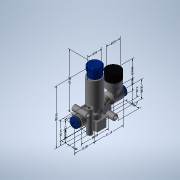
# Autodesk Inventor part: 8086003 VRPA-CM-Q4-E---(0_high)
Saved by Autodesk Inventor 2021 (Build 250183000, 183)
## iProperties
Created: 2026-04-20
Part Number: 8086003 VRPA-CM-Q4-E---(0_high)
Material: Generic
Catalog Web Link: www.3dfindit.com
Description: VRPA-C-Pressure regulator
Vendor: FESTO
Document SubType Name: Modeling
Designer: psAdmin
Manufacturer: FESTO
Mass: 23 g
Surface Area: 88.8725 cm^2
Volume: 16.5409 cm^3
Density: 1 g/cm^3
Appearance: PSOLRGB-176-176-176
Category: PARTsolutions
Company: FESTO
Title: 8086003 VRPA-CM-Q4-E
Author: Cadenas PARTsolutions
Comments: Pressure regulator
PSOL_IDENT_0: {$CADENAS_DATA/23d-libs/festo/parts/v/vrpa/vrpa_c.prj},206 {VTYP=3D},{NB=8086003 VRPA-CM-Q4-E---(0_h
PSOL_IDENT_1: igh)},{LINA=8086003 VRPA-CM-Q4-E},{NN=VRPA-C},{DATE=02.05.2025 13:44:11},{GEOMDATE=11.03.2025 15:31:
PSOL_IDENT_2: 33},{VERSION=},{LINEID=40},{WBVAR=HUB,LODLEVEL},{WBNUMERIC=HUB}  {NB=8086003 VRPA-CM-Q4-E---(0_high)
PSOL_IDENT_3: },{LINA=8086003 VRPA-CM-Q4-E},{KT=DUMMY},{TNR=8086003},{TYP=VRPA-CM-Q4-E},{HUB=0.000},{LODDEST=mecha
PSOL_IDENT_4: nical},{LODLEVEL=high},{LODLEVELX='high', 'High', 'medium', 'Medium','low','Low'},{P1=4},{P1N=4.000}
PSOL_IDENT_5: ,{P2=11.500},{P3=15.000},{L1=11.600},{L2=22.200},{L3=31.200},{L4=13.000},{L5=18.800},{L6L=59.000},{L
PSOL_IDENT_6: 6U=61.600},{L7=15.000},{L8=9.000},{L9=15.000},{L10=30.000},{L11=4.200},{L12=17.000},{L13=43.300},{L1
PSOL_IDENT_7: 4=10.100},{L15=20.200},{L16=10.200},{L17=24.500},{B=1.000},{VERS=2},{CNSMASSEXACT=0.023},{HUB1=2.600
PSOL_IDENT_8: },{GTIN=4052568458676},{REACH=Ja},{REACHSVHC=Ja},{REACHHAZSUBS=7439-92-1},{REACHSCIP=fd64103f-23d5-4
PSOL_IDENT_9: 69d-8662-7263eb37ed8b},{REACHVALDATE=05.03.2025}
NB: 8086003 VRPA-CM-Q4-E---(0_high)
NN: VRPA-C
NT: Pressure regulator
NBSYN: $TNR. $TYP.---($HUB._$LODLEVEL.)
LINA: 8086003 VRPA-CM-Q4-E
CATALOG: Festo
TNR: 8086003
TYP: VRPA-CM-Q4-E
HUB: 0
LODLEVEL: High
P1: 4
P2: 11.5
P3: 15
L1: 11.6
L2: 22.2
L3: 31.2
L4: 13
L5: 18.8
L6L: 59
L6U: 61.6
L7: 15
L8: 9
L9: 15
L10: 30
L11: 4.2
L12: 17
L13: 43.3
L14: 10.1
L15: 20.2
L16: 10.2
L17: 24.5
B: 1
CNSMASSEXACT: 0.023
GTIN: 4052568458676
REACH: Yes
REACHSVHC: Yes
REACHHAZSUBS: 7439-92-1
REACHVALDATE: 05.03.2025
SUPPLIER: FESTO
ARTICLENO: 8086003 VRPA-CM-Q4-E---(0_high)
BOMINFO: 8086003 VRPA-CM-Q4-E
CREATOR: CADENAS GmbH
Autodesk Inventor part; units mm, degrees
ref_plane "YZ Plane" through (0, 0, 0) normal (1, 0, 0) x (0, 1, 0)
ref_plane "XZ Plane" through (0, 0, 0) normal (0, 1, 0) x (-1, 0, 0)
ref_plane "XY Plane" through (0, 0, 0) normal (0, 0, 1) x (1, 0, 0)
sketch "Sketch_1" plane through (0, 0, 0) normal (0, 1, 0) x (-1, 0, 0)
  line L0 (7.5, 5) -> (4.899, 5)
  arc A0 (4.899, 5) -> (-4.899, 5) centre (0, 0) ccw
  line L1 (-4.899, 5) -> (-7.5, 5)
  line L2 (-7.5, 5) -> (-7.5, -5)
  line L3 (-7.5, -5) -> (-4.899, -5)
  arc A1 (-4.899, -5) -> (4.899, -5) centre (0, 0) ccw
  line L4 (4.899, -5) -> (7.5, -5)
  line L5 (7.5, -5) -> (7.5, 5)
  constraints: 12 end point, 4 point on circle, 2 centre point
extrude "Extrusion1" add sketch "Sketch_1" along normal blind 9.5
sketch "Sketch_2" plane through (0, 0, 0) normal (1, 0, 0) x (0, 1, 0)
  line L0 (0, 0) -> (59, 0)
  line L1 (59, 0) -> (59, -6)
  line L2 (59, -6) -> (57.8757, -6.9774)
  arc A0 (57.5477, -7.1) -> (57.8757, -6.9774) centre (57.5477, -6.6) ccw
  line L3 (57.5477, -7.1) -> (54.2, -7.1)
  arc A1 (53.7, -6.6) -> (54.2, -7.1) centre (54.2, -6.6) ccw
  line L4 (53.7, -6.6) -> (53.7, -6.3)
  line L5 (53.7, -6.3) -> (48.1, -6.3)
  line L6 (48.1, -6.3) -> (48.1, -2.5)
  line L7 (48.1, -2.5) -> (48, -2.5)
  line L8 (48, -2.5) -> (48, -7)
  arc A2 (47.5, -7.5) -> (48, -7) centre (47.5, -7) ccw
  line L9 (47.5, -7.5) -> (19.8, -7.5)
  arc A3 (19.3, -7) -> (19.8, -7.5) centre (19.8, -7) ccw
  line L10 (19.3, -7) -> (19.3, -5)
  arc A4 (19.3, -5) -> (18.8, -4.5) centre (18.8, -5) ccw
  line L11 (18.8, -4.5) -> (15.8071, -4.5)
  arc A5 (15.8071, -4.5) -> (15.4536, -4.6464) centre (15.8071, -5) ccw
  line L12 (15.4536, -4.6464) -> (14.2464, -5.8536)
  arc A6 (13.8929, -6) -> (14.2464, -5.8536) centre (13.8929, -5.5) ccw
  line L13 (13.8929, -6) -> (0, -6)
  line L14 (0, -6) -> (0, 0)
  line L15 (0, 0) -> (59, 0)
  constraints: 32 end point, 14 point on circle, 7 centre point
revolve "Revolution1" add sketch "Sketch_2" angle 360 about axis through (0, 0, 0) along (0, -1, 0)
sketch "Sketch_3" plane through (0, 59, 0) normal (0, 1, 0) x (1, 0, 0)
  circle A0 centre (0, 0) radius 8
  arc A1 (-7.0753, 0.5917) -> (-7.0753, -0.5917) centre (0, 0) ccw
  arc A2 (-7.0753, -0.5917) -> (-6.577, -1.05) centre (-6.577, -0.55) ccw
  line L0 (-6.577, -1.05) -> (-6.2119, -1.05)
  arc A3 (-6.2119, -1.05) -> (-5.9046, -2.1966) centre (0, 0) ccw
  line L1 (-5.9046, -2.1966) -> (-6.2209, -2.3792)
  arc A4 (-6.2209, -2.3792) -> (-6.4232, -3.0253) centre (-5.9709, -2.8122) ccw
  arc A5 (-6.4232, -3.0253) -> (-5.8316, -4.0501) centre (0, 0) ccw
  arc A6 (-5.8316, -4.0501) -> (-5.1709, -4.1978) centre (-5.4209, -3.7648) ccw
  line L2 (-5.1709, -4.1978) -> (-4.8546, -4.0153)
  arc A7 (-4.8546, -4.0153) -> (-4.0153, -4.8546) centre (0, 0) ccw
  line L3 (-4.0153, -4.8546) -> (-4.1978, -5.1709)
  arc A8 (-4.1978, -5.1709) -> (-4.0501, -5.8316) centre (-3.7648, -5.4209) ccw
  arc A9 (-4.0501, -5.8316) -> (-3.0253, -6.4232) centre (0, 0) ccw
  arc A10 (-3.0253, -6.4232) -> (-2.3792, -6.2209) centre (-2.8122, -5.9709) ccw
  line L4 (-2.3792, -6.2209) -> (-2.1966, -5.9046)
  arc A11 (-2.1966, -5.9046) -> (-1.05, -6.2119) centre (0, 0) ccw
  line L5 (-1.05, -6.2119) -> (-1.05, -6.577)
  arc A12 (-1.05, -6.577) -> (-0.5917, -7.0753) centre (-0.55, -6.577) ccw
  arc A13 (-0.5917, -7.0753) -> (0.5917, -7.0753) centre (0, 0) ccw
  arc A14 (0.5917, -7.0753) -> (1.05, -6.577) centre (0.55, -6.577) ccw
  line L6 (1.05, -6.577) -> (1.05, -6.2119)
  arc A15 (1.05, -6.2119) -> (2.1966, -5.9046) centre (0, 0) ccw
  line L7 (2.1966, -5.9046) -> (2.3792, -6.2209)
  arc A16 (2.3792, -6.2209) -> (3.0253, -6.4232) centre (2.8122, -5.9709) ccw
  arc A17 (3.0253, -6.4232) -> (4.0501, -5.8316) centre (0, 0) ccw
  arc A18 (4.0501, -5.8316) -> (4.1978, -5.1709) centre (3.7648, -5.4209) ccw
  line L8 (4.1978, -5.1709) -> (4.0153, -4.8546)
  arc A19 (4.0153, -4.8546) -> (4.8546, -4.0153) centre (0, 0) ccw
  line L9 (4.8546, -4.0153) -> (5.1709, -4.1978)
  arc A20 (5.1709, -4.1978) -> (5.8316, -4.0501) centre (5.4209, -3.7648) ccw
  arc A21 (5.8316, -4.0501) -> (6.4232, -3.0253) centre (0, 0) ccw
  arc A22 (6.4232, -3.0253) -> (6.2209, -2.3792) centre (5.9709, -2.8122) ccw
  line L10 (6.2209, -2.3792) -> (5.9046, -2.1966)
  arc A23 (5.9046, -2.1966) -> (6.2119, -1.05) centre (0, 0) ccw
  line L11 (6.2119, -1.05) -> (6.577, -1.05)
  arc A24 (6.577, -1.05) -> (7.0753, -0.5917) centre (6.577, -0.55) ccw
  arc A25 (7.0753, -0.5917) -> (7.0753, 0.5917) centre (0, 0) ccw
  arc A26 (7.0753, 0.5917) -> (6.577, 1.05) centre (6.577, 0.55) ccw
  line L12 (6.577, 1.05) -> (6.2119, 1.05)
  arc A27 (6.2119, 1.05) -> (5.9046, 2.1966) centre (0, 0) ccw
  line L13 (5.9046, 2.1966) -> (6.2209, 2.3792)
  arc A28 (6.2209, 2.3792) -> (6.4232, 3.0253) centre (5.9709, 2.8122) ccw
  arc A29 (6.4232, 3.0253) -> (5.8316, 4.0501) centre (0, 0) ccw
  arc A30 (5.8316, 4.0501) -> (5.1709, 4.1978) centre (5.4209, 3.7648) ccw
  line L14 (5.1709, 4.1978) -> (4.8546, 4.0153)
  arc A31 (4.8546, 4.0153) -> (4.0153, 4.8546) centre (0, 0) ccw
  line L15 (4.0153, 4.8546) -> (4.1978, 5.1709)
  arc A32 (4.1978, 5.1709) -> (4.0501, 5.8316) centre (3.7648, 5.4209) ccw
  arc A33 (4.0501, 5.8316) -> (3.0253, 6.4232) centre (0, 0) ccw
  arc A34 (3.0253, 6.4232) -> (2.3792, 6.2209) centre (2.8122, 5.9709) ccw
  line L16 (2.3792, 6.2209) -> (2.1966, 5.9046)
  arc A35 (2.1966, 5.9046) -> (1.05, 6.2119) centre (0, 0) ccw
  line L17 (1.05, 6.2119) -> (1.05, 6.577)
  arc A36 (1.05, 6.577) -> (0.5917, 7.0753) centre (0.55, 6.577) ccw
  arc A37 (0.5917, 7.0753) -> (-0.5917, 7.0753) centre (0, 0) ccw
  arc A38 (-0.5917, 7.0753) -> (-1.05, 6.577) centre (-0.55, 6.577) ccw
  line L18 (-1.05, 6.577) -> (-1.05, 6.2119)
  arc A39 (-1.05, 6.2119) -> (-2.1966, 5.9046) centre (0, 0) ccw
  line L19 (-2.1966, 5.9046) -> (-2.3792, 6.2209)
  arc A40 (-2.3792, 6.2209) -> (-3.0253, 6.4232) centre (-2.8122, 5.9709) ccw
  arc A41 (-3.0253, 6.4232) -> (-4.0501, 5.8316) centre (0, 0) ccw
  arc A42 (-4.0501, 5.8316) -> (-4.1978, 5.1709) centre (-3.7648, 5.4209) ccw
  line L20 (-4.1978, 5.1709) -> (-4.0153, 4.8546)
  arc A43 (-4.0153, 4.8546) -> (-4.8546, 4.0153) centre (0, 0) ccw
  line L21 (-4.8546, 4.0153) -> (-5.1709, 4.1978)
  arc A44 (-5.1709, 4.1978) -> (-5.8316, 4.0501) centre (-5.4209, 3.7648) ccw
  arc A45 (-5.8316, 4.0501) -> (-6.4232, 3.0253) centre (0, 0) ccw
  arc A46 (-6.4232, 3.0253) -> (-6.2209, 2.3792) centre (-5.9709, 2.8122) ccw
  line L22 (-6.2209, 2.3792) -> (-5.9046, 2.1966)
  arc A47 (-5.9046, 2.1966) -> (-6.2119, 1.05) centre (0, 0) ccw
  line L23 (-6.2119, 1.05) -> (-6.577, 1.05)
  arc A48 (-6.577, 1.05) -> (-7.0753, 0.5917) centre (-6.577, 0.55) ccw
  constraints: 96 point on circle, 49 centre point, 48 end point
extrude "Extrusion2" cut sketch "Sketch_3" against normal blind 5.3
sketch "Sketch_6" plane through (0, 0, 0) normal (0, 0, 1) x (1, 0, 0)
  line L0 (-4.35, 5.4) -> (-4.35, 4.2)
  line L1 (-4.35, 4.2) -> (3.15, 4.2)
  line L2 (3.15, 4.2) -> (3.15, 5.4)
  line L3 (3.15, 5.4) -> (0, 5.4)
  line L4 (0, 5.4) -> (0, 17.05)
  line L5 (0, 17.05) -> (-1.2, 17.05)
  line L6 (-1.2, 17.05) -> (-1.2, 5.4)
  line L7 (-1.2, 5.4) -> (-4.35, 5.4)
  constraints: 16 end point
extrude "Extrusion3" add sketch "Sketch_6" against normal blind 18
sketch "Sketch_15" plane through (3.15, 5.4, -18) normal (0, 0, -1) x (-1, 0, 0)
  line L0 (0, -3) -> (7.5, -3)
  line L1 (7.5, -3) -> (7.5, 0)
  line L2 (7.5, 0) -> (4.35, 0)
  line L3 (4.35, 0) -> (4.35, -2)
  line L4 (4.35, -2) -> (3.15, -2)
  line L5 (3.15, -2) -> (3.15, 0)
  line L6 (3.15, 0) -> (0, 0)
  line L7 (0, 0) -> (0, -3)
  constraints: 16 end point
extrude "Extrusion4" cut sketch "Sketch_15" against normal blind 5
sketch "Sketch_18" plane through (0, 0, 0) normal (1, 0, 0) x (0, 1, 0)
  line L0 (18.8, -31.2) -> (18.8, 0)
  line L1 (18.8, 0) -> (21.3, 0)
  line L2 (21.3, 0) -> (21.3, -8.36)
  line L3 (21.3, -8.36) -> (22.3, -9.36)
  line L4 (22.3, -9.36) -> (22.3, -13.5)
  line L5 (22.3, -13.5) -> (24.55, -15.75)
  line L6 (24.55, -15.75) -> (24.55, -25)
  line L7 (24.55, -25) -> (24.4452, -27)
  line L8 (24.4452, -27) -> (23.55, -27)
  line L9 (23.55, -27) -> (23.85, -27.3)
  line L10 (23.85, -27.3) -> (23.85, -27.6)
  line L11 (23.85, -27.6) -> (23.55, -27.9)
  line L12 (23.55, -27.9) -> (23.85, -28.2)
  line L13 (23.85, -28.2) -> (23.85, -28.6)
  line L14 (23.85, -28.6) -> (23.55, -28.9)
  line L15 (23.55, -28.9) -> (21.7, -28.9)
  line L16 (21.7, -28.9) -> (21.7, -29.2)
  arc A0 (21.7, -29.2) -> (22.2, -29.7) centre (22.2, -29.2) ccw
  line L17 (22.2, -29.7) -> (23.85, -29.7)
  line L18 (23.85, -29.7) -> (23.85, -31.2)
  line L19 (23.85, -31.2) -> (18.8, -31.2)
  line L20 (18.8, -31.2) -> (18.8, 0)
  constraints: 42 end point, 2 point on circle, 1 centre point
revolve "Revolution2" add sketch "Sketch_18" angle 360 about axis through (0, 18.8, -31.2) along (0, 0, -1)
sketch "Sketch_4" plane through (-1, 0, 0) normal (1, 0, 0) x (0, 0, -1)
  line L0 (0, 13.0001) -> (-22.2, 13.0001)
  line L1 (-22.2, 13.0001) -> (-22.2, 18.0501)
  line L2 (-22.2, 18.0501) -> (-20.7, 18.0501)
  line L3 (-20.7, 18.0501) -> (-20.7, 16.4001)
  arc A0 (-20.7, 16.4001) -> (-20.2, 15.9001) centre (-20.2, 16.4001) ccw
  line L4 (-20.2, 15.9001) -> (-19.9, 15.9001)
  line L5 (-19.9, 15.9001) -> (-19.9, 17.7501)
  line L6 (-19.9, 17.7501) -> (-19.6, 18.0501)
  line L7 (-19.6, 18.0501) -> (-19.2, 18.0501)
  line L8 (-19.2, 18.0501) -> (-18.9, 17.7501)
  line L9 (-18.9, 17.7501) -> (-18.6, 18.0501)
  line L10 (-18.6, 18.0501) -> (-18.3, 18.0501)
  line L11 (-18.3, 18.0501) -> (-18, 17.7501)
  line L12 (-18, 17.7501) -> (-18, 18.6453)
  line L13 (-18, 18.6453) -> (-16, 18.7501)
  line L14 (-16, 18.7501) -> (-11.25, 18.7501)
  line L15 (-11.25, 18.7501) -> (-9, 16.5001)
  line L16 (-9, 16.5001) -> (-6.66, 16.5001)
  line L17 (-6.66, 16.5001) -> (-5.66, 15.5001)
  line L18 (-5.66, 15.5001) -> (0, 15.5001)
  line L19 (0, 15.5001) -> (0, 13.0001)
  line L20 (0, 13.0001) -> (-22.2, 13.0001)
  constraints: 42 end point, 2 point on circle, 1 centre point
revolve "Revolution3" add sketch "Sketch_4" angle 360 about axis through (-1, 13.0001, 0) along (0, 0, -1)
sketch "Sketch_5" plane through (0, 4.2, 0) normal (0, 1, 0) x (1, 0, 0)
  line L0 (7.5, 15) -> (-7.5, 15)
  line L1 (-7.5, 15) -> (-7.5, 18)
  line L2 (-7.5, 18) -> (7.5, 18)
  line L3 (7.5, 18) -> (7.5, 15)
  line L4 (7.5, 15) -> (-7.5, 15)
  constraints: 10 end point
revolve "Revolution4" add sketch "Sketch_5" angle 360 about axis through (7.5, 4.2, -15) along (1, 0, 0)
sketch "Sketch9" plane through (7.5, 4.2, -15) normal (1, 0, 0) x (0, 0, -1)
  point P0 (0, 0)
hole "Hole1" at (7.5, 4.2, -15) direction (-1, 0, 0) diameter 3.3 depth 15
sketch "Sketch_9" plane through (-4.5, 0, 0) normal (1, 0, 0) x (0, 0, -1)
  line L0 (10.1, 0) -> (10.1, 24.5)
  line L1 (10.1, 24.5) -> (13, 24.5)
  line L2 (13, 24.5) -> (13, 0)
  line L3 (13, 0) -> (10.1, 0)
  line L4 (10.1, 0) -> (10.1, 24.5)
  constraints: 10 end point
revolve "Revolution5" add sketch "Sketch_9" angle 360 about axis through (-4.5, 0, -10.1) along (0, -1, 0)
sketch "Sketch11" plane through (-4.5, 0, -10.1) normal (0, -1, 0) x (1, 0, 0)
  point P0 (0, 0)
hole "Hole2" at (-4.5, 0, -10.1) direction (0, 1, 0) diameter 3.3 depth 24.5
sketch "Sketch_16" plane through (0, 24, 0) normal (0, 1, 0) x (1, 0, 0)
  line L0 (-2.2, -2.15) -> (-2.2, -15.1)
  line L1 (-2.2, -15.1) -> (-1, -15.1)
  line L2 (-1, -15.1) -> (-1, -13)
  line L3 (-1, -13) -> (4.5, -13)
  line L4 (4.5, -13) -> (4.5, -11.8)
  line L5 (4.5, -11.8) -> (-1, -11.8)
  line L6 (-1, -11.8) -> (-1, -8.4)
  line L7 (-1, -8.4) -> (4.5, -8.4)
  line L8 (4.5, -8.4) -> (4.5, -7.2)
  line L9 (4.5, -7.2) -> (0, -7.2)
  line L10 (0, -7.2) -> (0, -2.15)
  line L11 (0, -2.15) -> (-2.2, -2.15)
  constraints: 24 end point
extrude "Extrusion5" add sketch "Sketch_16" against normal blind 12.25
sketch "Sketch_11" plane through (4.5, 0, 0) normal (1, 0, 0) x (0, 0, -1)
  line L0 (-10.1, 0) -> (-10.1, 24.5)
  line L1 (-10.1, 24.5) -> (-7.2, 24.5)
  line L2 (-7.2, 24.5) -> (-7.2, 0)
  line L3 (-7.2, 0) -> (-10.1, 0)
  line L4 (-10.1, 0) -> (-10.1, 24.5)
  constraints: 10 end point
revolve "Revolution6" add sketch "Sketch_11" angle 360 about axis through (4.5, 0, 10.1) along (0, -1, 0)
sketch "Sketch14" plane through (4.5, 0, 10.1) normal (0, -1, 0) x (1, 0, 0)
  point P0 (0, 0)
hole "Hole3" at (4.5, 0, 10.1) direction (0, 1, 0) diameter 3.3 depth 24.5
sketch "Sketch_13" plane through (0, 21.2, 0) normal (0, 1, 0) x (1, 0, 0)
  line L0 (7.5, -15) -> (-7.5, -15)
  line L1 (-7.5, -15) -> (-7.5, -12)
  line L2 (-7.5, -12) -> (7.5, -12)
  line L3 (7.5, -12) -> (7.5, -15)
  line L4 (7.5, -15) -> (-7.5, -15)
  constraints: 10 end point
revolve "Revolution7" add sketch "Sketch_13" angle 360 about axis through (7.5, 21.2, 15) along (1, 0, 0)
sketch "Sketch16" plane through (7.5, 21.2, 15) normal (1, 0, 0) x (0, 0, -1)
  point P0 (0, 0)
hole "Hole4" at (7.5, 21.2, 15) direction (-1, 0, 0) diameter 3.3 depth 15
sketch "Sketch_21" plane through (0, 0, 0) normal (1, 0, 0) x (0, 1, 0)
  line L0 (18.8, -20.3) -> (43.3, -20.3)
  line L1 (43.3, -20.3) -> (43.3, -27.6)
  arc A0 (43.1, -27.8) -> (43.3, -27.6) centre (43.1, -27.6) ccw
  line L2 (43.1, -27.8) -> (35.3, -27.8)
  line L3 (35.3, -27.8) -> (35.3, -27.75)
  line L4 (35.3, -27.75) -> (32.5, -27.75)
  line L5 (32.5, -27.75) -> (32.3, -27.55)
  line L6 (32.3, -27.55) -> (32.3, -27.8)
  line L7 (32.3, -27.8) -> (28.3, -27.8)
  arc A1 (27.8, -27.3) -> (28.3, -27.8) centre (28.3, -27.3) ccw
  line L8 (27.8, -27.3) -> (27.8, -25.8)
  arc A2 (27.8, -25.8) -> (27.3, -25.3) centre (27.3, -25.8) ccw
  line L9 (27.3, -25.3) -> (18.8, -25.3)
  line L10 (18.8, -25.3) -> (18.8, -20.3)
  line L11 (18.8, -20.3) -> (43.3, -20.3)
  constraints: 24 end point, 6 point on circle, 3 centre point
revolve "Revolution8" add sketch "Sketch_21" angle 360 about axis through (0, 18.8, -20.3) along (0, -1, 0)
sketch "Sketch_7" plane through (0, 0, 0) normal (1, 0, 0) x (0, 1, 0)
  line L0 (18.8, -34.2) -> (18.8, -19.6)
  line L1 (18.8, -19.6) -> (20.8, -19.6)
  line L2 (20.8, -19.6) -> (20.8, -30.8954)
  arc A0 (20.8, -30.8954) -> (21.1521, -31.1908) centre (21.1, -30.8954) ccw
  line L3 (21.1521, -31.1908) -> (23.6847, -30.7442)
  arc A1 (23.6847, -30.7442) -> (23.85, -30.5473) centre (23.65, -30.5473) ccw
  line L4 (23.85, -30.5473) -> (23.85, -34.2)
  line L5 (23.85, -34.2) -> (18.8, -34.2)
  line L6 (18.8, -34.2) -> (18.8, -19.6)
  constraints: 14 end point, 4 point on circle, 2 centre point
revolve "Revolution9" cut sketch "Sketch_7" angle 360 about axis through (0, 18.8, -34.2) along (0, 0, -1)
sketch "Sketch_17" plane through (-1, 0, 0) normal (1, 0, 0) x (0, 0, -1)
  line L0 (-10.6, 13.0001) -> (-25.2, 13.0001)
  line L1 (-25.2, 13.0001) -> (-25.2, 18.0501)
  line L2 (-25.2, 18.0501) -> (-21.5473, 18.0501)
  arc A0 (-21.5473, 18.0501) -> (-21.7442, 17.8848) centre (-21.5473, 17.8501) ccw
  line L3 (-21.7442, 17.8848) -> (-22.1908, 15.3522)
  arc A1 (-22.1908, 15.3522) -> (-21.8954, 15.0001) centre (-21.8954, 15.3001) ccw
  line L4 (-21.8954, 15.0001) -> (-10.6, 15.0001)
  line L5 (-10.6, 15.0001) -> (-10.6, 13.0001)
  line L6 (-10.6, 13.0001) -> (-25.2, 13.0001)
  constraints: 14 end point, 4 point on circle, 2 centre point
revolve "Revolution10" cut sketch "Sketch_17" angle 360 about axis through (-1, 13.0001, 10.6) along (0, 0, -1)
sketch "Sketch_19" plane through (0, 48, 0) normal (0, 1, 0) x (1, 0, 0)
  line L0 (-12.5, -8.5) -> (12.5, -8.5)
  line L1 (12.5, -8.5) -> (12.5, 8.5)
  line L2 (12.5, 8.5) -> (-12.5, 8.5)
  line L3 (-12.5, 8.5) -> (-12.5, -8.5)
  line L4 (-9.5, -7) -> (9.5, -7)
  line L5 (9.5, -7) -> (9.5, 7)
  line L6 (9.5, 7) -> (-9.5, 7)
  line L7 (-9.5, 7) -> (-9.5, -7)
  constraints: 16 end point
extrude "Extrusion6" cut sketch "Sketch_19" against normal blind 2
body "Solid1"
